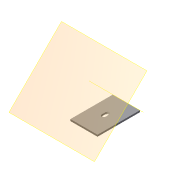
# Autodesk Inventor part: 00_Comar_Dichroic_16x25x0.2
Saved by Autodesk Inventor 2019 (Build 230136000, 136)
## iProperties
Created: 2019-08-10
Part Number: 00_Comar_Dichroic_16x25x0.2
Material: Generic
Document SubType Name: Modeling
Designer: diederichbenedict
Density: 1 g/cm^3
Appearance: Default
Author: diederichbenedict
Autodesk Inventor part; units mm, degrees
ref_plane "YZ Plane" through (0, 0, 0) normal (1, 0, 0) x (0, 1, 0)
ref_plane "XZ Plane" through (0, 0, 0) normal (0, 1, 0) x (-1, 0, 0)
ref_plane "XY Plane" through (0, 0, 0) normal (0, 0, 1) x (1, 0, 0)
sketch "Sketch1" plane through (0, 0, 0) normal (0, 1, 0) x (-1, 0, 0)
  line L0 (0, 0) -> (16, 0)
  line L1 (16, 0) -> (16, -25)
  line L2 (16, -25) -> (0, -25)
  line L3 (0, -25) -> (0, 0)
  circle A0 centre (8, -12.5) radius 1.1261
  dimension "d0" = 16
  dimension "d1" = 25
  constraints: 8 end point, 2 parallel, 1 centre point, 1 horizontal, 1 perpendicular
  measures "d0" distance of L1.end L2.end
  measures "d1" distance of L0.end L1.end
extrude "Extrusion1" add sketch "Sketch1" along normal blind 1
ref_plane "Work Plane1" through (16.9, 36.305, -11.9513) normal (0, 0.7071, 0.7071) x (-1, 0, 0)
sketch "Sketch2" plane through (16.9, 36.305, -11.9513) normal (0, 0.7071, 0.7071) x (-1, 0, 0)
  ellipse E0 centre (24.9, 24.5764) end of major axis (23.7739, 24.5764) minor radius 0.7963 projected
  circle A0 centre (24.9, 24.9) radius 1.1798
  ellipse E1 centre (24.9, 25.2835) end of major axis (23.7739, 25.2835) minor radius 0.7963 projected
  point P0 (16.9, 34.1223)
  dimension "d4" = 0.3236
  constraints: 1 centre point, 3 other
  measures "d4" distance of point (24.9, 24.576) A0.centre
extrude "Extrusion2" cut sketch "Sketch2" against normal through all contours E0 E1 A0 | E0 A0 E1 | E1 A0 E0 | E0 E1 | E0 A0 | E1 A0 E0 picked at (24.9476, 23.7672)
ref_plane "Work Plane2" through (0, 1, -25) normal (0, 0.7071, -0.7071) x (1, 0, 0)
sketch "Sketch3" plane through (0, 1, -25) normal (0, 0.7071, -0.7071) x (1, 0, 0)
  arc A0 (-7.287, -8.2225) -> (-8.713, -8.2225) centre (-8, -9.1624) ccw projected
  ellipse E0 centre (-8, -8.8388) end of major axis (-6.8739, -8.8388) minor radius 0.7963 (-6.8748, -8.8079) -> (-7.287, -8.2225) ccw projected
  arc A1 (-9.1252, -8.8079) -> (-6.8748, -8.8079) centre (-8, -9.1624) ccw projected
  ellipse E1 centre (-8, -8.8388) end of major axis (-6.8739, -8.8388) minor radius 0.7963 (-8.713, -8.2225) -> (-9.1252, -8.8079) ccw projected
  line L0 (-16, -17.6777) -> (0, -17.6777) projected
  line L1 (0, -17.6777) -> (0, 0) projected
  line L2 (0, 0) -> (-16, 0) projected
  line L3 (-16, 0) -> (-16, -17.6777) projected
  line L4 (0, 0.7071) -> (0, -16.9706) construction
  line L5 (-16, 0) -> (-16, -17.6777) construction
  line L6 (-16, -17.6777) -> (0, -17.6777) construction
  line L7 (-16, -17.6777) -> (0, -17.6777) construction
  arc A2 (-9.1252, -8.8079) -> (-6.8748, -8.8079) centre (-8, -9.1624) ccw construction
  arc A3 (-7.287, -8.2225) -> (-8.713, -8.2225) centre (-8, -9.1624) ccw construction
  arc A4 (-6.8747, -8.1025) -> (-9.1253, -8.1025) centre (-8, -7.7482) ccw construction
  line L8 (-16, 0.7071) -> (0, 0.7071) projected
  line L9 (0, 0.7071) -> (-16, -17.6777)
  line L10 (0, -17.6777) -> (0, 0) projected
  line L11 (0, -17.6777) -> (-16, 0.7071)
  circle A5 centre (-8, -8.4853) radius 1.1706
  point P0 (-8, -8.928)
  constraints: 6 end point, 1 centre point, 1 collinear, 1 midpoint, 6 other
extrude "Extrusion3" cut sketch "Sketch3" against normal blind 25.4 contours E0 A5 L11 L9 A0 | A0 L9 A5 E0 | L9 L11 A0 | A0 L11 A5 L9 | L11 L9 A5 E1 A0 | A0 E1 A5 L11 | L11 A5 L9
body "Solid1"
